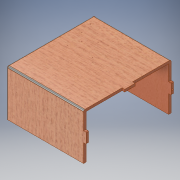
# Autodesk Inventor part: OpticalDeviceObjectPart
Saved by Autodesk Inventor 2017 (Build 210142000, 142)
## iProperties
Created: 2019-04-01
Part Number: OpticalDeviceObjectPart
Material: Generic
Document SubType Name: Modeling
Designer: 625311
Density: 1 g/cm^3
Appearance: Walnut - Natural Polished
Author: 625311
Autodesk Inventor part; units mm, degrees
ref_plane "YZ Plane" through (0, 0, 0) normal (1, 0, 0) x (0, 1, 0)
ref_plane "XZ Plane" through (0, 0, 0) normal (0, 1, 0) x (-1, 0, 0)
ref_plane "XY Plane" through (0, 0, 0) normal (0, 0, 1) x (1, 0, 0)
sketch "Sketch1" plane through (0, 0, 0) normal (0, 1, 0) x (-1, 0, 0)
  line L0 (0, 0) -> (-150, 0)
  line L1 (0, -170) -> (0, 0)
  line L2 (0, -170) -> (-150, -170)
  line L3 (-150, -170) -> (-150, -95)
  line L4 (-150, -95) -> (-155, -95)
  line L5 (-155, -95) -> (-155, -75)
  line L6 (-155, -75) -> (-150, -75)
  line L7 (-150, -75) -> (-150, 0)
  dimension "d28" = 150
  dimension "d29" = 170
  dimension "d30" = 5
  dimension "d31" = 5
  dimension "d32" = 75
  dimension "d33" = 75
  dimension "d34" = 20
  dimension "d35" = 150
  constraints: 16 end point, 4 perpendicular, 2 horizontal, 2 vertical, 1 point on line
  measures "d28" distance of L0.start L0.end
  measures "d29" distance of L1.start L0.start
  measures "d30" distance of L3.end L4.end
  measures "d31" distance of L5.end L6.end
  measures "d32" distance of L2.end L3.end
  measures "d33" distance of L6.end L0.end
  measures "d34" distance of L4.end L5.end
  measures "d35" distance between parallel lines of L7 L1
extrude "Extrusion1" add sketch "Sketch1" along normal blind 4.7625
sketch "Sketch2" plane through (0, 0, 0) normal (0, -1, 0) x (1, 0, 0)
  line L0 (0, 0) -> (150, 0) projected
  line L1 (0, 0) -> (4.7625, 0)
  line L2 (150, -170) -> (0, -170) projected
  line L3 (0, 0) -> (0, -170)
  line L4 (0, -170) -> (4.7625, -170)
  line L5 (4.7625, -170) -> (4.7625, 0)
  point P0 (0, -90)
  point P1 (4.7625, -90)
  dimension "d10" = 90
  dimension "d11" = 4.7625
  constraints: 8 end point, 2 point on line, 1 collinear, 1 perpendicular, 1 vertical
  measures "d10" distance of L1.end point (4.763, -90)
  measures "d11" distance of L1.end L0.start
extrude "Extrusion2" add sketch "Sketch2" along normal blind 85.2375
sketch "Sketch3" plane through (0, 0, 0) normal (0, -1, 0) x (1, 0, 0)
  line L0 (150, -95) -> (150, -170) projected
  line L1 (150, -170) -> (150, -165.2375)
  line L2 (150, -165.2375) -> (4.7625, -165.2375)
  line L3 (4.7625, 0) -> (4.7625, -170) projected
  line L4 (150, -170) -> (4.7625, -170) projected
  line L5 (4.7625, -170) -> (4.7625, -165.2375)
  line L6 (150, -170) -> (4.7625, -170)
  line L7 (150, -170) -> (150, -165.2375)
  point P0 (0, 0)
  dimension "d36" = 4.7625
  constraints: 10 end point, 3 perpendicular, 2 point on line, 1 collinear
  measures "d36" distance of L0.end L1.end
sketch "Sketch4" plane through (0, 0, 0) normal (0, -1, 0) x (1, 0, 0)
  line L0 (150, 0) -> (150, -35) projected
  line L1 (150, 0) -> (150, -4.7625)
  line L2 (150, -4.7625) -> (4.7625, -4.7625)
  line L3 (4.7625, -85.2375) -> (4.7625, 0) projected
  line L4 (4.7625, 0) -> (150, 0)
  line L5 (4.7625, 0) -> (150, 0) projected
  line L6 (4.7625, -4.7625) -> (4.7625, 0)
  point P0 (0, 0)
  dimension "d17" = 4.7625
  constraints: 8 end point, 2 point on line, 1 parallel, 1 perpendicular, 1 vertical
  measures "d17" distance of L1.end L0.start
extrude "Extrusion4" add sketch "Sketch4" along normal blind 85.2375
sketch "Sketch6" plane through (0, 4.7625, 0) normal (0, 0, 1) x (1, 0, 0)
  line L0 (150, -4.7625) -> (150, -90) projected
  line L1 (150, -4.7625) -> (150, -90) projected
  line L2 (150, -90) -> (0, -90) projected
  line L3 (0, 0) -> (150, 0) projected
  line L4 (150, -55) -> (155, -55)
  line L5 (155, -55) -> (155, -35)
  line L6 (155, -35) -> (150, -35)
  line L7 (150, -35) -> (150, -55)
  point P0 (0, -4.7625)
  point P1 (150, -31.3995)
  dimension "d90" = 20
  dimension "d91" = 5
  dimension "d92" = 35
  dimension "d93" = 35
  constraints: 8 end point, 2 parallel, 2 point on line, 1 horizontal, 1 perpendicular
  measures "d90" distance of L4.end L5.end
  measures "d91" distance of L4.start L4.end
  measures "d92" distance from line of L0.end L4
  measures "d93" distance between parallel lines of L3 L6
extrude "Extrusion6" add sketch "Sketch6" against normal blind 4.7625
extrude "Extrusion7" add sketch "Sketch3" along normal blind 85.2375
sketch "Sketch7" plane through (150, 4.7625, -170) normal (0, 0, -1) x (-1, 0, 0)
  line L0 (0, -4.7625) -> (0, -90) projected
  line L1 (0, -55) -> (-5, -55)
  line L2 (-5, -55) -> (-5, -35)
  line L3 (-5, -35) -> (0, -35)
  line L4 (0, -35) -> (0, -55)
  line L5 (150, -90) -> (0, -90) projected
  line L6 (0, 0) -> (150, 0) projected
  point P0 (150, -4.7625)
  point P1 (-5, -31.3995)
  dimension "d74" = 20
  dimension "d75" = 5
  dimension "d76" = 35
  dimension "d77" = 35
  constraints: 8 end point, 2 parallel, 1 horizontal, 1 perpendicular, 1 point on line
  measures "d74" distance of L1.end L2.end
  measures "d75" distance of L1.start L1.end
  measures "d76" distance between parallel lines of L5 L1
  measures "d77" distance between parallel lines of L6 L3
extrude "Extrusion8" add sketch "Sketch7" against normal blind 4.7625
fillet "Fillet3" radius 3 1 edges at (0, 4.7625, -85)
fillet "Fillet4" radius 3 6 edges at (0.8787, 3.8838, -170) (0, -41.7375, -170) (76.5, 4.7625, -170) (0.8787, 3.8838, 0) (0, -41.7375, 0) (76.5, 4.7625, 0)
hole "Hole3" at (155, 2.4466, -85.2501) direction (-1, 0, 0) diameter 2.5 depth 5 tip angle 118
hole "Hole4" at (155, -42.3344, -167.7364) direction (-1, 0, 0) diameter 2.5 depth 5 tip angle 118
fillet "Fillet5" radius 1 2 edges at (155, -50.2375, -167.6188) (155, -30.2375, -167.6188)
fillet "Fillet6" radius 1 2 edges at (155, -50.2375, -2.3813) (155, -30.2375, -2.3813)
body "Solid1"
